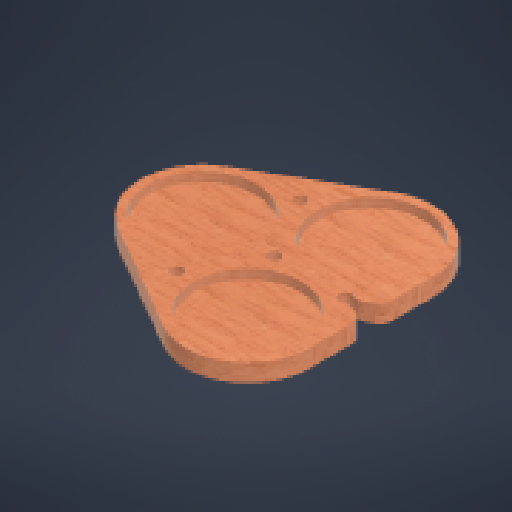
# Autodesk Inventor part: BOTTOM_PLATE_WEIGHTS_TREBUCHET
Saved by Autodesk Inventor 2026.2 (Build 302298010, 298A)
## iProperties
Created: 2026-02-19
Part Number: BOTTOM_PLATE_WEIGHTS_TREBUCHET
Material: Wood (Oak)
Document SubType Name: Modeling
Designer: 4aida
Density: 0.76 g/cm^3
Appearance: White Oak - Natural Medium Gloss
Mass: 58.4633 g
Surface Area: 302.014 cm^2
Volume: 76.9253 cm^3
Author: 4aida
Autodesk Inventor part; units mm, degrees
ref_plane "YZ Plane" through (0, 0, 0) normal (1, 0, 0) x (0, 1, 0)
ref_plane "XZ Plane" through (0, 0, 0) normal (0, 1, 0) x (-1, 0, 0)
ref_plane "XY Plane" through (0, 0, 0) normal (0, 0, 1) x (1, 0, 0)
sketch "Sketch1" plane through (0, 0, 0) normal (0, 1, 0) x (-1, 0, 0)
  line L0 (54.6051, -28.5788) -> (-2.5526, -61.5788)
  line L1 (-52.0526, -33) -> (-52.0526, 33)
  line L2 (-2.5526, 61.5788) -> (54.6051, 28.5788)
  circle A0 centre (38.1051, 0) radius 33 construction
  circle A1 centre (-19.0526, 33) radius 33 construction
  circle A2 centre (-19.0526, -33) radius 33 construction
  arc A3 (54.6051, -28.5788) -> (54.6051, 28.5788) centre (38.1051, 0) ccw
  arc A4 (-52.0526, -33) -> (-2.5526, -61.5788) centre (-19.0526, -33) ccw
  arc A5 (-2.5526, 61.5788) -> (-52.0526, 33) centre (-19.0526, 33) ccw
  circle A6 centre (0, 0) radius 3.175
  line L3 (-52.0526, -4.875) -> (-48.6526, -4.875)
  line L4 (-48.6526, -4.875) -> (-40.9371, -1.3266)
  line L5 (-40.9371, 1.3266) -> (-48.6526, 4.875)
  line L6 (-48.6526, 4.875) -> (-52.0526, 4.875)
  arc A7 (-40.9371, -1.3266) -> (-40.9371, 1.3266) centre (-38.0526, 0) ccw
  line L7 (-40.9371, -1.3266) -> (-38.0526, 0) construction
  line L8 (-38.0526, 0) -> (-40.9371, 1.3266) construction
  arc A8 (21.6175, -34.7893) -> (19.3197, -36.1159) centre (19.0263, -32.9545) ccw
  arc A9 (19.3197, 36.1159) -> (21.6175, 34.7893) centre (19.0263, 32.9545) ccw
  circle A10 centre (19.0263, 32.9545) radius 3.175
  circle A11 centre (19.0263, -32.9545) radius 3.175
  point P0 (-52.0526, 0)
  point P1 (-52.0526, 0)
  point P2 (21.6175, -34.7893)
  point P3 (21.6175, 34.7893)
  dimension "d1" = 66
  dimension "d14" = 6.35
  dimension "d15" = 9.75
  dimension "d16" = 3.4
  dimension "d18" = 10.6
  dimension "d20" = 6.35
  dimension "d23" = 360
  constraints: 18 end point, 18 point on circle, 10 centre point, 9 tangent, 5 coincident, 4 concentric, 2 collinear, 2 equal length, 2 horizontal alignment, 2 midpoint, 2 point on line, 1 horizontal, 1 perpendicular, 1 vertical, 23 other
  measures "d1" diameter of A0
  measures "d14" diameter of A6
  measures "d15" distance between parallel lines of L6 L3
  measures "d16" distance of L3.start L3.end
  measures "d18" horizontal distance of L3.end point (-38.053, 0)
  measures "d20" diameter of A7
extrude "Extrusion1" add sketch "Sketch1" along normal blind 9.525 contours L0 A4 L1 L3 L4 A7 L5 L6 A5 L2 A3
sketch "Sketch2" plane through (0, 9.525, 0) normal (0, 1, 0) x (1, 0, 0)
  circle A0 centre (19.0526, -33) radius 28.575
  circle A1 centre (-38.1051, 0) radius 28.575
  circle A2 centre (19.0526, 33) radius 28.575
  circle A3 centre (19.0526, 33) radius 33
  circle A4 centre (-38.1051, 0) radius 33
  circle A5 centre (19.0526, -33) radius 33
  line L0 (-54.6051, -28.5788) -> (2.5526, -61.5788) projected
  line L1 (2.5526, 61.5788) -> (-54.6051, 28.5788) projected
  line L2 (52.0526, -33) -> (52.0526, 33) projected
  point P0 (0, 0)
  point P1 (-99.3426, -2.7496)
  point P2 (47.2901, -87.408)
  point P3 (47.2901, 87.408)
  point P4 (-99.3426, 2.7496)
  point P5 (52.0526, -84.6584)
  point P6 (52.0526, 84.6584)
  dimension "d5" = 57.15
  constraints: 9 tangent, 6 centre point, 3 coincident, 2 equal radius
  measures "d5" diameter of A0
extrude "Extrusion2" cut sketch "Sketch2" against normal blind 5 contours A0 | A1 | A2
fillet "Fillet2" radius 6.35 4 edges at (52.0526, 4.7625, -4.875) (52.0526, 4.7625, 4.875) (40.9371, 4.7625, -1.3266) (40.9371, 4.7625, 1.3266)
body "Solid1"
